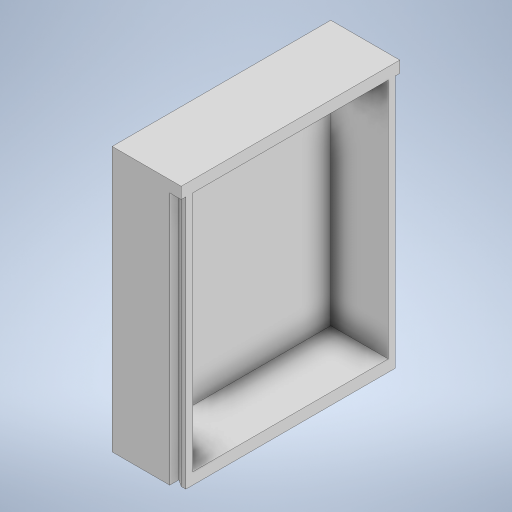
# Autodesk Inventor part: carcasa_pcb
Saved by Autodesk Inventor 2024.3 (Build 283343000, 343)
## iProperties
Created: 2025-07-17
Part Number: carcasa_pcb
Material: Genérico
Document SubType Name: Modeling
Designer: Damian
Density: 1 g/cm^3
Appearance: Valor por defecto
Author: Damian
Autodesk Inventor part; units mm, degrees
ref_plane "YZ Plane" through (0, 0, 0) normal (1, 0, 0) x (0, 1, 0)
ref_plane "XZ Plane" through (0, 0, 0) normal (0, 1, 0) x (-1, 0, 0)
ref_plane "XY Plane" through (0, 0, 0) normal (0, 0, 1) x (1, 0, 0)
sketch "Boceto1" plane through (0, 0, 0) normal (1, 0, 0) x (0, 1, 0)
  line L0 (0, 0) -> (105, 0)
  line L1 (105, 0) -> (105, -85)
  line L2 (105, -85) -> (0, -85)
  line L3 (0, -85) -> (0, 0)
  line L4 (110, 5) -> (-5, 5)
  line L5 (-5, 5) -> (-5, -90)
  line L6 (-5, -90) -> (110, -90)
  line L7 (110, -90) -> (110, 5)
  point P0 (105, -42.5)
  dimension "d0" = 85
  dimension "d1" = 105
  dimension "d2" = 5
  dimension "d3" = 5
  dimension "d4" = 5
  dimension "d5" = 5
  constraints: 16 end point, 4 parallel, 2 horizontal, 2 perpendicular, 1 midpoint
  measures "d0" distance of L0.end L1.end
  measures "d1" distance of L1.end L2.end
  measures "d2" distance from line of point (105, -42.5) L7
  measures "d3" distance between parallel lines of L6 L2
  measures "d4" distance between parallel lines of L0 L4
  measures "d5" distance between parallel lines of L5 L3
extrude "Extrusión1" add sketch "Boceto1" along normal blind 30
extrude "Extrusión2" add sketch "Boceto1" along normal blind 5 contours L0 L1 L2 L3
sketch "Boceto2" plane through (0, -5, -90) normal (0, -1, 0) x (1, 0, 0)
  line L0 (0, 0) -> (30, 0) projected
  line L1 (30, 0) -> (30, 2)
  line L2 (30, 0) -> (30, 95) projected
  line L3 (28, 2) -> (25, 4)
  line L4 (25, 4) -> (25, 0)
  line L5 (25, 0) -> (30, 0)
  line L6 (30, 2) -> (28, 2)
  line L7 (37.2923, 47.5) -> (-11.4995, 47.5) construction
  line L8 (30, 95) -> (30, 93)
  line L9 (28, 93) -> (25, 91)
  line L10 (25, 91) -> (25, 95)
  line L11 (25, 95) -> (30, 95)
  line L12 (30, 93) -> (28, 93)
  point P0 (0, 90)
  point P1 (30, 47.5)
  point P2 (25, 0)
  dimension "d10" = 2
  dimension "d11" = 2
  dimension "d12" = 4
  dimension "d13" = 5
  dimension "d14" = 0
  constraints: 22 end point, 4 symmetric about line, 2 horizontal, 1 midpoint, 1 parallel, 1 perpendicular, 1 point on line
  measures "d10" distance of L1.end L3.start
  measures "d11" distance of L0.end L1.end
  measures "d12" distance of L3.end L4.end
  measures "d13" distance of L4.end L0.end
  measures "d14" distance from line of point (30, 47.5) L7
extrude "Extrusión3" cut sketch "Boceto2" against normal blind 110
